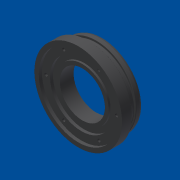
# Autodesk Inventor part: Deckel_unten_BFA_35_30_10
Saved by Autodesk Inventor 2018.3 (Build 223284000, 284)
## iProperties
Created: 2016-11-15
Part Number: Deckel_unten_BFA_35_30_10
Material: PVC, hart
Document SubType Name: Modeling
Designer: stud_brinkmann
Mass: 40.76 g
Surface Area: 134.143 cm^2
Volume: 31.5969 cm^3
Density: 1.29 g/cm^3
Appearance: Glatt - weiß
Author: stud_brinkmann
Autodesk Inventor part; units mm, degrees
ref_plane "YZ Plane" through (0, 0, 0) normal (1, 0, 0) x (0, 1, 0)
ref_plane "XZ Plane" through (0, 0, 0) normal (0, 1, 0) x (-1, 0, 0)
ref_plane "XY Plane" through (0, 0, 0) normal (0, 0, 1) x (1, 0, 0)
sketch "Skizze2" plane through (0, 0, 0) normal (1, 0, 0) x (0, 1, 0)
  line L0 (0, 0) -> (18.8, 0)
  line L1 (3.3, 18) -> (14.3, 18)
  line L2 (18.8, 31.354) -> (17.3, 31.9)
  line L3 (17.3, 31.9) -> (14.3, 31.9)
  line L4 (14.3, 31.9) -> (14.3, 30.15)
  line L5 (14.3, 30.15) -> (10.8, 30.15)
  line L6 (10.8, 30.15) -> (10.8, 31.9)
  line L7 (10.8, 31.9) -> (7.8, 31.9)
  line L8 (7.8, 31.9) -> (7.8, 35)
  line L9 (7.8, 35) -> (0, 35)
  line L10 (0, 35) -> (0, 31.5)
  line L11 (0, 31.5) -> (2.5, 31.5)
  line L12 (2.5, 31.5) -> (2.5, 25)
  line L13 (2.5, 25) -> (4.8, 25)
  line L14 (4.8, 25) -> (4.8, 21)
  line L15 (4.8, 21) -> (3.3, 21)
  line L16 (3.3, 21) -> (3.3, 18)
  line L17 (18.8, 31.354) -> (18.8, 27.5)
  line L18 (18.8, 27.5) -> (14.3, 27.5)
  line L19 (14.3, 27.5) -> (14.3, 18)
  dimension "d5" = 36
  dimension "d10" = 20
  dimension "d11" = 60.3
  dimension "d12" = 63.8
  dimension "d15" = 3
  dimension "d16" = 1.5
  dimension "d17" = 4
  dimension "d19" = 2.3
  dimension "d20" = 63
  dimension "d26" = 70
  dimension "d28" = 2.5
  dimension "d33" = 11
  dimension "d34" = 1.5
  dimension "d35" = 4.5
  dimension "d36" = 8
  dimension "d37" = 11
  dimension "d53" = 55
  dimension "d54" = 4.5
  constraints: 40 end point, 13 perpendicular, 2 horizontal, 2 point on line, 2 vertical, 2 vertical alignment, 1 parallel
  measures "d5" diameter of L1 L0
  measures "d10" angle of L3 L2
  measures "d11" diameter of L5 L0
  measures "d12" diameter of L3 L0
  measures "d15" distance of L15.end L1.start
  measures "d16" distance of L14.end L15.end
  measures "d17" distance of L13.end L14.end
  measures "d19" distance of L12.end L13.end
  measures "d20" diameter of L11 L0
  measures "d26" diameter of L9 L0
  measures "d28" distance of L10.end L11.end
  measures "d33" distance between parallel lines of L16 L19
  measures "d34" distance from line of L2.end L17
  measures "d35" distance between parallel lines of L4 L17
  measures "d36" distance between parallel lines of L6 L17
  measures "d37" distance between parallel lines of L8 L17
  measures "d53" diameter of L18 L0
  measures "d54" distance of L17.end L18.end
revolve "Umdrehung1" add sketch "Skizze2" angle 360 about axis through (0, 0, 0) along (0, 1, 0)
fillet "Rundung1" radius 0.3 4 edges at (0, 10.8, -30.15) (0, 14.3, -30.15) (0, 10.8, -31.9) (0, 14.3, -31.9)
sketch "Skizze5" plane through (0, 2.5, 0) normal (0, -1, 0) x (1, 0, 0)
  line L0 (0, 0) -> (35, 0) construction
  circle A0 centre (0, 0) radius 35 construction
  point P0 (28.15, 0)
  point P1 (14.075, 24.3786)
  point P2 (-14.075, 24.3786)
  point P3 (-28.15, 0)
  point P4 (-14.075, -24.3786)
  point P5 (14.075, -24.3786)
  dimension "d58" = 28.15
  dimension "d61" = 360
  constraints: 2 end point, 1 horizontal, 1 horizontal alignment, 1 point on line, 8 other
  measures "d58" distance of point (28.15, 0) L0.start
hole "Bohrung3" at (28.15, 2.5, 0) at (14.075, 2.5, 24.3786) at (-14.075, 2.5, 24.3786) at (-28.15, 2.5, 0) at (-14.075, 2.5, -24.3786) at (14.075, 2.5, -24.3786) direction (0, 1, 0) diameter 2.459 depth 6.5 tip angle 118 thread size "M3x0.5" class "6H" standard "ISO Metric profile"
sketch "Skizze6" plane through (0, 14.3, 0) normal (0, 1, 0) x (1, 0, 0)
  circle A0 centre (0, 0) radius 22.65
  point P0 (0, 23.65)
  point P1 (20.45, -9.7376)
  point P2 (-20.45, -9.7376)
  dimension "d72" = 45.3
  dimension "d70" = 23.65
  dimension "d71" = 40.9
  constraints: 1 coincident, 3 other
  measures "d70" distance of point (0, 23.65) point (0, 0)
  measures "d71" distance of point (-20.45, -9.738) point (20.45, -9.738)
hole "Bohrung5" at (0, 14.3, -23.65) at (20.45, 14.3, 9.7376) at (-20.45, 14.3, 9.7376) direction (0, -1, 0) diameter 2.5 depth 6 tip angle 118
thread "Gewinde1" size "M3x0.5" class "6H" standard "ANSI Metric M Profile" full length
thread "Gewinde2" size "M3x0.5" class "6H" standard "ANSI Metric M Profile" full length
thread "Gewinde3" size "M3x0.5" class "6H" standard "ANSI Metric M Profile" full length
equation "\"d36\" = d35 + ORing1"
equation "\"ORing1\" = 3.5"
